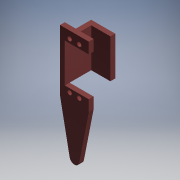
# Autodesk Inventor part: Lower_leg
Saved by Autodesk Inventor 2017 (Build 210142000, 142)
## iProperties
Part Number: Lower_leg
Material: Generic
Document SubType Name: Modeling
Designer: alex-
Appearance: Chestnut
Author: alex-
Autodesk Inventor part; units mm, degrees
ref_plane "YZ Plane" through (0, 0, 0) normal (1, 0, 0) x (0, 1, 0)
ref_plane "XZ Plane" through (0, 0, 0) normal (0, 1, 0) x (-1, 0, 0)
ref_plane "XY Plane" through (0, 0, 0) normal (0, 0, 1) x (1, 0, 0)
sketch "Sketch1" plane through (0, 0, 0) normal (0, 0, 1) x (1, 0, 0)
  point P0 (0, 0)
sketch "Sketch2" plane through (0, 0, 0) normal (0, 0, 1) x (1, 0, 0)
  line L0 (-15, 113.5) -> (15, 113.5)
  line L1 (15, 113.5) -> (15, 50)
  line L2 (15, 50) -> (-15, 50) construction
  line L3 (-15, 50) -> (-15, 113.5)
  circle A0 centre (0, 0) radius 5 construction
  line L4 (-15, 50) -> (-4.9047, -0.9714)
  line L5 (15, 50) -> (4.9047, -0.9714)
  arc A1 (-4.9047, -0.9714) -> (4.9047, -0.9714) centre (0, 0) ccw
  point P0 (0, 50)
  dimension "d0" = 30
  dimension "d1" = 63.5
  dimension "d2" = 10
  dimension "d3" = 50
  constraints: 12 end point, 4 point on circle, 2 centre point, 2 coincident, 2 parallel, 1 concentric, 1 equal length, 1 horizontal, 1 midpoint, 1 perpendicular, 1 tangent, 1 vertical alignment
  measures "d0" distance of L0.start L0.end
  measures "d1" distance between parallel lines of L2 L0
  measures "d2" diameter of A0
  measures "d3" distance from line of L2 A1.centre
extrude "Extrusion1" add sketch "Sketch2" along normal blind 5
sketch "Sketch3" plane through (0, 0, 5) normal (0, 0, 1) x (1, 0, 0)
  line L0 (-10, 108.5) -> (10, 108.5) construction
  line L1 (10, 108.5) -> (10, 55) construction
  line L2 (10, 55) -> (-10, 55) construction
  line L3 (-10, 55) -> (-10, 108.5) construction
  line L4 (15, 113.5) -> (-15, 113.5) construction
  circle A0 centre (-5, 106) radius 2.25
  circle A1 centre (5, 106) radius 2.25
  circle A2 centre (-5, 57.5) radius 2.25
  circle A3 centre (5, 57.5) radius 2.25
  line L5 (-10, 61.5) -> (10, 61.5)
  line L6 (10, 61.5) -> (10, 102)
  line L7 (10, 102) -> (-10, 102)
  line L8 (-10, 102) -> (-10, 61.5)
  line L9 (0, 108.5) -> (0, 55) construction
  point P0 (0, 0)
  point P1 (-10, 81.75)
  point P2 (10, 81.75)
  point P3 (0, 81.75)
  dimension "d6" = 20
  dimension "d7" = 53.5
  dimension "d8" = 5
  dimension "d9" = 4.5
  dimension "d11" = 2.75
  dimension "d12" = 2.5
  dimension "d13" = 2.75
  dimension "d14" = 2.5
  dimension "d15" = 40.5
  constraints: 18 end point, 7 midpoint, 4 centre point, 4 parallel, 3 equal radius, 3 horizontal alignment, 3 vertical alignment, 2 horizontal, 2 perpendicular
  measures "d6" distance of L0.start L0.end
  measures "d7" distance of L2.end L0.start
  measures "d8" distance between parallel lines of L0 L4
  measures "d9" diameter of A0
  measures "d11" distance edge to line of A0 L3
  measures "d12" distance from line of A0.centre L0
  measures "d13" distance edge to line of A1 L1
  measures "d14" distance from line of L2 A2.centre
  measures "d15" distance between parallel lines of L5 L7
extrude "Extrusion2" cut sketch "Sketch3" against normal up to next
sketch "Sketch4" plane through (15, 50, 0) normal (1, 0, 0) x (0, 0, -1)
  line L0 (-5, 52) -> (0, 52)
  line L1 (0, 52) -> (0, 11.5)
  line L2 (0, 11.5) -> (-5, 11.5)
  line L3 (-5, 11.5) -> (-5, 52)
  line L4 (-5, 52) -> (0, 52) projected
  line L5 (-5, 11.5) -> (0, 11.5) projected
  line L6 (0, 63.5) -> (0, 0) projected
  point P0 (0, -50)
  point P1 (-2.5, 52)
  point P2 (-2.5, 11.5)
  point P3 (0, 31.75)
  constraints: 8 end point, 6 midpoint, 2 parallel, 1 horizontal, 1 perpendicular
extrude "Extrusion3" cut sketch "Sketch4" against normal up to surface (5 mm away)
sketch "Sketch8" plane through (0, 0, 0) normal (0, 0, -1) x (-1, 0, 0)
  line L0 (15, 102) -> (10, 102)
  line L1 (10, 102) -> (10, 61.5)
  line L2 (10, 61.5) -> (15, 61.5)
  line L3 (15, 61.5) -> (15, 102)
  line L4 (15, 50) -> (15, 113.5) projected
  line L5 (10, 102) -> (10, 61.5) projected
  point P0 (0, 0)
  point P1 (15, 81.75)
  point P2 (10, 81.75)
  point P3 (12.5, 61.5)
  point P4 (12.5, 102)
  constraints: 8 end point, 6 midpoint, 2 horizontal alignment, 2 parallel, 1 horizontal, 1 perpendicular
extrude "Extrusion6" add sketch "Sketch8" along normal blind 27.5
sketch "Sketch9" plane through (-10, 61.5, 5) normal (1, 0, 0) x (0, 0, -1)
  line L0 (27.5, 40.5) -> (32.5, 40.5)
  line L1 (32.5, 40.5) -> (32.5, 0)
  line L2 (32.5, 0) -> (27.5, 0)
  line L3 (27.5, 0) -> (27.5, 40.5)
  line L4 (32.5, 40.5) -> (32.5, 0) projected
  line L5 (5, 40.5) -> (32.5, 40.5) projected
  line L6 (5, 0) -> (32.5, 0) projected
  point P0 (5, -61.5)
  point P1 (32.5, 20.25)
  point P2 (30, 40.5)
  point P3 (30, 0)
  dimension "d27" = 5
  constraints: 8 end point, 4 midpoint, 2 parallel, 2 point on line, 1 horizontal, 1 perpendicular
  measures "d27" distance of L0.start L0.end
extrude "Extrusion7" add sketch "Sketch9" along normal blind 20
equation "\"d0\" = s_depth + 2 * b_mat_thickness"
equation "\"d1\" = 2 * s_land + s_width + 2 * b_mat_thickness"
equation "\"d4\" = b_mat_thickness"
equation "\"d6\" = s_depth"
equation "\"d7\" = s_width + 2 * s_land"
equation "\"d8\" = b_mat_thickness"
equation "\"d9\" = s_hole_dia"
equation "\"d11\" = s_hole_side_dist"
equation "\"d12\" = s_hole_front_dist"
equation "\"d13\" = s_hole_side_dist"
equation "\"d14\" = s_hole_front_dist"
equation "\"d15\" = s_width"
equation "\"d16\" = b_mat_thickness"
equation "\"d25\" = -s_land_dist_top + s_height - s_land_thickness"
equation "\"d27\" = b_mat_thickness"
equation "\"d28\" = s_depth"
equation "\"s_depth\" = 20"
equation "\"b_mat_thickness\" = 5"
equation "\"s_land\" = 6.5"
equation "\"s_width\" = 40.5"
equation "\"s_hole_dia\" = 4.5"
equation "\"s_hole_side_dist\" = 2.75"
equation "\"s_hole_front_dist\" = 2.5"
equation "\"s_land_dist_top\" = 8"
equation "\"s_height\" = 38"
equation "\"s_land_thickness\" = 2.5"
body "Solid1"
